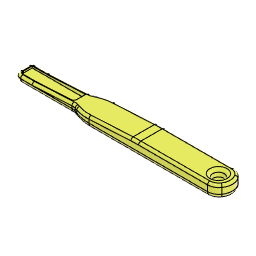
Nozzle Brush A3 (Autodesk Fusion 360 design; units mm, degrees)
Autodesk Fusion 360 part; units mm, degrees
sketch "Sketch1" plane through (0, 0, 0) normal (0, 0, 1) x (1, 0, 0)
  arc A0 (-18.55, -2.05) -> (-16.55, -4.05) centre (-16.55, -2.05) ccw
  line L0 (-16.55, -4.05) -> (16.55, -4.05)
  arc A1 (16.55, -4.05) -> (18.55, -2.05) centre (16.55, -2.05) ccw
  line L1 (18.55, -2.05) -> (18.55, 4.05)
  line L2 (18.55, 4.05) -> (-18.55, 4.05)
  line L3 (-18.55, 4.05) -> (-18.55, -2.05)
  line L4 (-20.55, 6.05) -> (28.55, 6.05)
  line L5 (28.55, 6.05) -> (28.55, -6.05)
  line L6 (28.55, -6.05) -> (-20.55, -6.05)
  line L7 (-20.55, -6.05) -> (-20.55, 6.05)
  line L8 (28.55, 9) -> (118.55, 9)
  line L9 (118.55, 9) -> (118.55, -9)
  line L10 (118.55, -9) -> (28.55, -9)
  line L11 (28.55, -9) -> (28.55, 9)
  line L12 (28.55, 9) -> (20.55, 6.05)
  line L13 (28.55, -9) -> (20.55, -6.05)
  arc A2 (118.55, -9) -> (118.55, 9) centre (114.8, 0) ccw
  circle A3 centre (114.8, 0) radius 4
  point P0 (28.55, 0)
  point P1 (28.55, 0)
  point P2 (124.55, 0)
  dimension "d1" = 2
  dimension "d2" = 2
  dimension "d3" = 10
  dimension "d4" = 2
  dimension "d5" = 18
  dimension "d6" = 90
  dimension "d7" = 2
  dimension "d8" = 6
  dimension "d33" = 8
  constraint horizontal L4
  constraint vertical L5
  constraint horizontal L6
  constraint vertical L7
  constraint horizontal L8
  constraint vertical L9
  constraint horizontal L10
  constraint vertical L11
  constraint midpoint L5 P1
  constraint midpoint L11 P1
  constraint coincident P1 P0
  constraint coincident L4 L12.end
  constraint coincident L6 L13.end
  constraint vertical L12.end L13.end
  constraint midpoint A2 P2
  constraint concentric A2 A3
  measures "d1" distance of L3 L7
  measures "d2" distance of L2 L4
  measures "d3" distance of L1 L11
  measures "d4" distance of L0 L6
  measures "d5" distance of L8.end L9.end
  measures "d6" distance of L8.start L8.end
  measures "d7" horizontal distance of L1.end L12.end
  measures "d8" distance of L9 P2
  measures "d33" diameter of A3
extrude "Extrude1" add sketch "Sketch1" along normal blind 4 contours A0 L0 A1 L1 L2 L3 | L4 L5 L6 L7 L11 | L4 L11 L12 | L5 L8 L9 L10 L11 A3 | L6 L11 L13 | L9 A2 A3
extrude "Extrude2" cut sketch "Sketch1" against normal blind 1.2 from surface at 4 contours A0 L0 A1 L1 L2 L3
extrude "Extrude3" add sketch "Sketch1" along normal blind 8 contours L5 L8 L9 L10 L11 A3 | L9 A2 A3
extrude "Extrude4" add 1 faces at (25.2167, -0.6833, 4) along direction (0, 0, 1) up to surface (4 mm away)
sketch "Sketch2" plane through (0, -6.05, 0) normal (0, -1, 0) x (1, 0, 0)
  line L0 (-20.55, 0) -> (20.55, 0)
  line L1 (20.55, 0) -> (20.55, 8)
  line L2 (20.55, 8) -> (-20.55, 8)
  line L3 (-20.55, 8) -> (-20.55, 0)
  line L4 (-18.55, 8) -> (-18.55, 2.8)
  line L5 (-18.55, 2.8) -> (18.55, 2.8)
  line L6 (18.55, 2.8) -> (18.55, 8)
  line L7 (18.55, 8) -> (-18.55, 8)
  line L8 (20.55, 0) -> (28.55, 0)
  line L9 (28.55, 0) -> (28.55, 8)
  line L10 (28.55, 8) -> (20.55, 8)
  line L11 (20.55, 8) -> (20.55, 0)
  line L12 (-8.55, 4) -> (28.55, 6)
  line L13 (28.55, 8) -> (65.65, 8)
  line L14 (65.65, 8) -> (28.55, 6)
  line L15 (-8.55, 4) -> (-20.55, 4)
  dimension "d52" = 2
  dimension "d55" = 1.2
  dimension "d56" = 10
  constraint coincident L9 L12.end
  constraint coincident L9.end L10.start
  constraint perpendicular L9 L13
  constraint collinear L12 L14
  constraint coincident L3 L15.end
  constraint horizontal L15
  measures "d52" distance of L9.end L12.end
  measures "d55" distance of L5 L15
  measures "d56" distance of L4 L12.start
extrude "Extrude5" cut sketch "Sketch2" along normal mid plane 100 contours L2 L3 L4 L15 | L1 L2 L6 L11 L12 | L1 L9 L10 L11 L12 | L2 L4 L6 L7 L12 L15 | L9 L13 L14
fillet "Fillet11" radius 8 2 edges at (20.55, -6.05, 2.7844) (20.55, 6.05, 2.7844)
fillet "Fillet12" radius 30 2 edges at (28.55, 9, 3) (28.55, -9, 3)
fillet "Fillet1" radius 4 1 edges at (-20.55, -6.05, 2)
fillet "Fillet2" radius 2 1 edges at (-20.55, 6.05, 2)
fillet "Fillet5" radius 8 2 edges at (118.55, -9, 2) (118.55, 9, 2)
fillet "Fillet14" radius 100 1 edges at (65.65, 0, 8)
fillet "Fillet7" radius 1.6 20 edges at (90.9431, -9, 8) (119.9394, -8.0912, 8) (124.55, 0, 8) (119.9394, 8.0912, 8) (90.9431, 9, 8) (5.286, 6.05, 4.7459) (20.5278, 6.1745, 5.5675) (22.7078, 6.8457, 5.6851) (28.6333, 8.5332, 6.0045) (49.7775, 9, 7.1443) (49.7775, -9, 7.1443) (28.6333, -8.5332, 6.0045) (22.7078, -6.8457, 5.6851) (20.5278, -6.1745, 5.5675) (5.286, -6.05, 4.7459) (-12.55, -6.05, 4) (-19.3784, -4.8784, 4) (-20.55, 1, 4) (-19.9642, 5.4642, 4) (-13.55, 6.05, 4)
chamfer "Chamfer1" distance 1.1 angle 40 1 faces at (59.5367, 0, 0)
fillet "Fillet13" radius 3 16 edges at (124.55, 0, 0.923) (119.9394, -8.0912, 0.923) (75.0706, -9, 0.923) (28.6333, -8.5332, 0.923) (22.7078, -6.8457, 0.923) (20.5278, -6.1745, 0.923) (1.286, -6.05, 0.923) (-19.3784, -4.8784, 0.923) (-20.55, 1, 0.923) (-19.9642, 5.4642, 0.923) (0.286, 6.05, 0.923) (20.5278, 6.1745, 0.923) (22.7078, 6.8457, 0.923) (28.6333, 8.5332, 0.923) (75.0706, 9, 0.923) (119.9394, 8.0912, 0.923)
fillet "Fillet9" radius 5 1 edges at (111.0707, -1.4465, 0.923)
fillet "Fillet15" radius 2 1 edges at (111.0707, 1.4465, 8)
equation "d10 = head_thick"
equation "d39 = body_thick"
equation "head_thick = 4 mm"
equation "body_thick = 8 mm"
